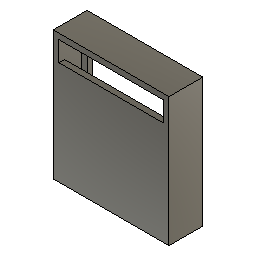
BME680_ENCLOSURE v4 (Autodesk Fusion 360 design; units mm, degrees)
Autodesk Fusion 360 part; units mm, degrees
(part 1 of 2)
sketch "Esboço1" plane through (0, 0.8, 0) normal (0, 1, 0) x (-1, 0, 0)
  line L0 (2.5, -12.15) -> (2.5, -7.85)
  arc A0 (3.5, -6.85) -> (2.5, -7.85) centre (3.5, -7.85) ccw
  line L1 (3.5, -6.85) -> (6.7, -6.85)
  line L2 (6.7, -6.85) -> (8.2, -5.35)
  line L3 (8.2, -5.35) -> (8.2, 6.85)
  line L4 (8.2, 6.85) -> (-8.2, 6.85)
  line L5 (-8.2, 6.85) -> (-8.2, -5.35)
  line L6 (-8.2, -5.35) -> (-6.7, -6.85)
  line L7 (-6.7, -6.85) -> (-3.5, -6.85)
  arc A1 (-2.5, -7.85) -> (-3.5, -6.85) centre (-3.5, -7.85) ccw
  line L8 (-2.5, -7.85) -> (-2.5, -12.15)
  line L9 (-2.5, -12.15) -> (2.5, -12.15)
  circle A2 centre (6.35, 5.85) radius 0.6
  circle A3 centre (-6.35, 5.85) radius 0.6
  circle A4 centre (-3.81, 5.85) radius 0.6
  circle A5 centre (-1.27, 5.85) radius 0.6
  circle A6 centre (1.27, 5.85) radius 0.6
  circle A7 centre (3.81, 5.85) radius 0.6
  spline S0 degree 3 poles (4.0814, 2.2721) (4.0816, 2.2764) (4.0819, 2.2848) (4.086, 2.2968) (4.0921, 2.3078) (4.1006, 2.3174) (4.1105, 2.3255) (4.1217, 2.3314) (4.1337, 2.3352) (4.1421, 2.3355) (4.1464, 2.3357) knots 0 0 0 0 0.126655 0.249859 0.371763 0.500453 0.628013 0.750799 0.873345 1 1 1 1
  spline S1 degree 3 poles (4.1464, 2.3357) (4.1506, 2.3355) (4.1588, 2.3352) (4.1707, 2.3313) (4.1818, 2.3255) (4.1915, 2.3174) (4.1998, 2.3078) (4.2056, 2.2966) (4.2095, 2.2845) (4.2098, 2.2761) (4.21, 2.2719) knots 0 0 0 0 0.12536 0.246668 0.370351 0.497111 0.625295 0.748978 0.872419 1 1 1 1
  line L10 (4.21, 2.2719) -> (4.21, 2.0201)
  spline S2 degree 3 poles (4.21, 2.0201) (4.2095, 2.0119) (4.2086, 1.9954) (4.2022, 1.9709) (4.1923, 1.9469) (4.1787, 1.9238) (4.1627, 1.9022) (4.1448, 1.8833) (4.1253, 1.8673) (4.1109, 1.8593) (4.1038, 1.8554) knots 0 0 0 0 0.120295 0.241539 0.367541 0.499794 0.632883 0.759219 0.880834 1 1 1 1
  line L11 (4.1038, 1.8554) -> (3.8515, 1.7288)
  spline S3 degree 3 poles (3.8515, 1.7288) (3.8401, 1.7233) (3.8175, 1.7125) (3.7819, 1.7011) (3.7455, 1.6941) (3.721, 1.6933) (3.7087, 1.6929) knots 0 0 0 0 0.255305 0.504536 0.751856 1 1 1 1
  spline S4 degree 3 poles (3.7087, 1.6929) (3.697, 1.6934) (3.6734, 1.6944) (3.6378, 1.702) (3.6016, 1.7137) (3.5784, 1.7251) (3.5665, 1.731) knots 0 0 0 0 0.234952 0.477147 0.731798 1 1 1 1
  line L12 (3.5665, 1.731) -> (3.3165, 1.8583)
  spline S5 degree 3 poles (3.3165, 1.8583) (3.3087, 1.8625) (3.2931, 1.8709) (3.2726, 1.8875) (3.2543, 1.9064) (3.2388, 1.9278) (3.2259, 1.951) (3.2168, 1.976) (3.2109, 2.0022) (3.2103, 2.0201) (3.21, 2.0292) knots 0 0 0 0 0.125475 0.2491 0.371934 0.496998 0.621836 0.746394 0.871303 1 1 1 1
  line L13 (3.21, 2.0292) -> (3.21, 2.2721)
  spline S6 degree 3 poles (3.21, 2.2721) (3.2102, 2.2764) (3.2106, 2.2848) (3.2143, 2.2968) (3.2205, 2.3077) (3.2287, 2.3174) (3.2384, 2.3255) (3.2493, 2.3314) (3.2612, 2.3352) (3.2694, 2.3355) (3.2736, 2.3357) knots 0 0 0 0 0.127946 0.25174 0.374887 0.503437 0.63056 0.752626 0.874282 1 1 1 1
  spline S7 degree 3 poles (3.2736, 2.3357) (3.2779, 2.3355) (3.2863, 2.3352) (3.2983, 2.3313) (3.3097, 2.3258) (3.3195, 2.3176) (3.3282, 2.3083) (3.3339, 2.2972) (3.3381, 2.2855) (3.3384, 2.2772) (3.3386, 2.273) knots 0 0 0 0 0.127432 0.250729 0.375227 0.50357 0.631371 0.752946 0.874787 1 1 1 1
  line L14 (3.3386, 2.273) -> (3.3386, 2.2071)
  line L15 (3.3386, 2.2071) -> (4.0814, 2.2071)
  line L16 (4.0814, 2.2071) -> (4.0814, 2.2721)
  spline S8 degree 3 poles (1.4325, 4.1605) (1.4397, 4.1654) (1.4537, 4.175) (1.4768, 4.1854) (1.5009, 4.1917) (1.5174, 4.1925) (1.5256, 4.1929) knots 0 0 0 0 0.259405 0.508544 0.754257 1 1 1 1
  spline S9 degree 3 poles (1.5256, 4.1929) (1.535, 4.1923) (1.5536, 4.1913) (1.5805, 4.1835) (1.6052, 4.1701) (1.6275, 4.1522) (1.6461, 4.1305) (1.6601, 4.1063) (1.6686, 4.0797) (1.6695, 4.0612) (1.67, 4.0518) knots 0 0 0 0 0.126245 0.24873 0.371883 0.501018 0.62976 0.75261 0.873755 1 1 1 1
  line L17 (1.67, 4.0518) -> (1.67, 3.729)
  spline S10 degree 3 poles (1.67, 3.729) (1.6694, 3.7192) (1.6683, 3.6993) (1.6576, 3.6704) (1.6412, 3.6426) (1.6227, 3.6208) (1.6054, 3.6047) (1.5915, 3.5937) (1.5766, 3.5849) (1.5613, 3.5772) (1.5452, 3.5713) (1.5284, 3.5674) (1.5109, 3.5648) (1.499, 3.5645) (1.493, 3.5643) knots 0 0 0 0 0.110459 0.223148 0.342644 0.474148 0.54296 0.6087 0.673406 0.737899 0.801293 0.865961 0.932005 1 1 1 1
  spline S11 degree 3 poles (1.493, 3.5643) (1.4886, 3.5646) (1.4799, 3.5651) (1.4673, 3.5689) (1.456, 3.5759) (1.4461, 3.5851) (1.4377, 3.5955) (1.4315, 3.6069) (1.4277, 3.619) (1.4273, 3.6273) (1.4271, 3.6315) knots 0 0 0 0 0.127348 0.250965 0.376177 0.506901 0.638364 0.760387 0.87927 1 1 1 1
  spline S12 degree 3 poles (1.4271, 3.6315) (1.4273, 3.6369) (1.4275, 3.6469) (1.4303, 3.6607) (1.4352, 3.6717) (1.4423, 3.6806) (1.4526, 3.6868) (1.4652, 3.6929) (1.4814, 3.6983) (1.4996, 3.7029) (1.5174, 3.7084) (1.5315, 3.7187) (1.54, 3.7328) (1.541, 3.7434) (1.5414, 3.7489) knots 0 0 0 0 0.089812 0.165231 0.230095 0.287663 0.349673 0.426046 0.519675 0.62936 0.736624 0.826058 0.910331 1 1 1 1
  line L18 (1.5414, 3.7489) -> (1.5414, 4.0431)
  spline S13 degree 3 poles (1.5414, 4.0431) (1.5414, 4.0462) (1.5412, 4.0518) (1.5382, 4.0588) (1.5333, 4.0637) (1.529, 4.0641) (1.5267, 4.0643) knots 0 0 0 0 0.323315 0.566859 0.773057 1 1 1 1
  spline S14 degree 3 poles (1.5267, 4.0643) (1.5233, 4.0639) (1.5155, 4.0631) (1.5091, 4.0583) (1.5055, 4.0556) knots 0 0 0 0 0.42835 1 1 1 1
  line L19 (1.5055, 4.0556) -> (0.9075, 3.5973)
  spline S15 degree 3 poles (0.9075, 3.5973) (0.9003, 3.5922) (0.8862, 3.5822) (0.8627, 3.5721) (0.8385, 3.5653) (0.8221, 3.5646) (0.8137, 3.5643) knots 0 0 0 0 0.261351 0.512303 0.754244 1 1 1 1
  spline S16 degree 3 poles (0.8137, 3.5643) (0.8045, 3.5647) (0.7861, 3.5656) (0.7596, 3.5735) (0.735, 3.5863) (0.7129, 3.6038) (0.6942, 3.6241) (0.68, 3.6461) (0.6716, 3.6698) (0.6705, 3.6861) (0.67, 3.6942) knots 0 0 0 0 0.130284 0.257797 0.385118 0.519315 0.651174 0.771096 0.886275 1 1 1 1
  line L20 (0.67, 3.6942) -> (0.67, 4.0283)
  spline S17 degree 3 poles (0.67, 4.0283) (0.6702, 4.0338) (0.6706, 4.0446) (0.6731, 4.0604) (0.6771, 4.0758) (0.6829, 4.0906) (0.6906, 4.1047) (0.6998, 4.1184) (0.7105, 4.1316) (0.727, 4.1479) (0.7492, 4.1656) (0.7781, 4.1813) (0.8085, 4.1911) (0.8294, 4.1923) (0.8399, 4.1929) knots 0 0 0 0 0.062642 0.124202 0.184472 0.245252 0.306591 0.369566 0.434735 0.502591 0.635605 0.760198 0.879447 1 1 1 1
  spline S18 degree 3 poles (0.8399, 4.1929) (0.8456, 4.1927) (0.8564, 4.1923) (0.8714, 4.1891) (0.8843, 4.1841) (0.8947, 4.1765) (0.9032, 4.1671) (0.9089, 4.1552) (0.9123, 4.1414) (0.9127, 4.1316) (0.9129, 4.1263) knots 0 0 0 0 0.152342 0.285545 0.405068 0.516839 0.624561 0.739342 0.861447 1 1 1 1
  spline S19 degree 3 poles (0.9129, 4.1263) (0.9127, 4.1222) (0.9123, 4.114) (0.9083, 4.1024) (0.9023, 4.0916) (0.8939, 4.0823) (0.8839, 4.0742) (0.8728, 4.0685) (0.8607, 4.0649) (0.8524, 4.0645) (0.8481, 4.0643) knots 0 0 0 0 0.123971 0.246778 0.365389 0.494204 0.623565 0.750071 0.871557 1 1 1 1
  spline S20 degree 3 poles (0.8481, 4.0643) (0.8447, 4.0641) (0.8381, 4.0638) (0.8286, 4.0612) (0.8201, 4.057) (0.8127, 4.0511) (0.8063, 4.044) (0.8019, 4.0357) (0.799, 4.0266) (0.7987, 4.0203) (0.7986, 4.017) knots 0 0 0 0 0.13474 0.258614 0.382591 0.505187 0.629267 0.752001 0.871073 1 1 1 1
  line L21 (0.7986, 4.017) -> (0.7986, 3.7125)
  spline S21 degree 3 poles (0.7986, 3.7125) (0.7986, 3.7095) (0.7987, 3.7043) (0.8021, 3.6977) (0.8076, 3.6931) (0.8122, 3.693) (0.8146, 3.6929) knots 0 0 0 0 0.302016 0.536312 0.750494 1 1 1 1
  spline S22 degree 3 poles (0.8146, 3.6929) (0.8176, 3.6933) (0.825, 3.6945) (0.8308, 3.6992) (0.8343, 3.702) knots 0 0 0 0 0.406145 1 1 1 1
  line L22 (0.8343, 3.702) -> (1.4325, 4.1605)
  line L23 (1.095, 3.1161) -> (0.8374, 2.983)
  spline S23 degree 3 poles (0.8374, 2.983) (0.8313, 2.9797) (0.8198, 2.9734) (0.8069, 2.9586) (0.7993, 2.9405) (0.7988, 2.9274) (0.7986, 2.9205) knots 0 0 0 0 0.262753 0.501306 0.739158 1 1 1 1
  line L24 (0.7986, 2.9205) -> (0.7986, 2.6875)
  spline S24 degree 3 poles (0.7986, 2.6875) (0.7984, 2.6832) (0.798, 2.6746) (0.7942, 2.6624) (0.7884, 2.6509) (0.78, 2.6409) (0.7705, 2.632) (0.7592, 2.6261) (0.7472, 2.6219) (0.7386, 2.6216) (0.7343, 2.6214) knots 0 0 0 0 0.126957 0.249782 0.372684 0.501426 0.62965 0.751659 0.873043 1 1 1 1
  spline S25 degree 3 poles (0.7343, 2.6214) (0.7299, 2.6216) (0.7214, 2.6219) (0.7094, 2.6261) (0.6981, 2.632) (0.6886, 2.6409) (0.6801, 2.6507) (0.6744, 2.6621) (0.6705, 2.6742) (0.6702, 2.6827) (0.67, 2.6871) knots 0 0 0 0 0.127439 0.249283 0.371755 0.500466 0.627999 0.751368 0.872561 1 1 1 1
  line L25 (0.67, 2.6871) -> (0.67, 2.927)
  spline S26 degree 3 poles (0.67, 2.927) (0.6703, 2.9348) (0.671, 2.9506) (0.6771, 2.9743) (0.6863, 2.9983) (0.6988, 3.022) (0.7133, 3.044) (0.729, 3.063) (0.7454, 3.0786) (0.7577, 3.086) (0.7635, 3.0895) knots 0 0 0 0 0.119524 0.243206 0.374508 0.515457 0.654341 0.779636 0.894797 1 1 1 1
  line L26 (0.7635, 3.0895) -> (1.0454, 3.235)
  spline S27 degree 3 poles (1.0454, 3.235) (1.0556, 3.2395) (1.0755, 3.2484) (1.1068, 3.2574) (1.1384, 3.2633) (1.1596, 3.264) (1.1702, 3.2643) knots 0 0 0 0 0.256397 0.506809 0.754246 1 1 1 1
  spline S28 degree 3 poles (1.1702, 3.2643) (1.1816, 3.2639) (1.2038, 3.2633) (1.2359, 3.2581) (1.2657, 3.2496) (1.2839, 3.2409) (1.2928, 3.2366) knots 0 0 0 0 0.269644 0.524554 0.766799 1 1 1 1
  line L27 (1.2928, 3.2366) -> (1.5718, 3.0895)
  spline S29 degree 3 poles (1.5718, 3.0895) (1.5782, 3.0857) (1.5913, 3.0779) (1.609, 3.0625) (1.6258, 3.0446) (1.6409, 3.0241) (1.6537, 3.0024) (1.6629, 2.9804) (1.669, 2.9587) (1.6697, 2.9443) (1.67, 2.9373) knots 0 0 0 0 0.119157 0.241726 0.37148 0.508504 0.645292 0.77099 0.888372 1 1 1 1
  line L28 (1.67, 2.9373) -> (1.67, 2.6853)
  spline S30 degree 3 poles (1.67, 2.6853) (1.6698, 2.681) (1.6695, 2.6726) (1.6657, 2.6606) (1.6598, 2.6496) (1.6515, 2.64) (1.6418, 2.6316) (1.6307, 2.6258) (1.6188, 2.622) (1.6106, 2.6216) (1.6064, 2.6214) knots 0 0 0 0 0.12765 0.251158 0.372942 0.501195 0.629448 0.753198 0.874572 1 1 1 1
  spline S31 degree 3 poles (1.6064, 2.6214) (1.6021, 2.6216) (1.5937, 2.622) (1.5817, 2.6258) (1.5705, 2.6316) (1.5606, 2.64) (1.552, 2.6496) (1.546, 2.6608) (1.5419, 2.6728) (1.5416, 2.6812) (1.5414, 2.6855) knots 0 0 0 0 0.126235 0.248374 0.370753 0.49928 0.627542 0.75097 0.873765 1 1 1 1
  line L29 (1.5414, 2.6855) -> (1.5414, 2.9299)
  spline S32 degree 3 poles (1.5414, 2.9299) (1.5413, 2.9348) (1.5409, 2.9446) (1.534, 2.9584) (1.5227, 2.9704) (1.5128, 2.9762) (1.5075, 2.9792) knots 0 0 0 0 0.230337 0.460431 0.709763 1 1 1 1
  line L30 (1.5075, 2.9792) -> (1.245, 3.1181)
  spline S33 degree 3 poles (1.245, 3.1181) (1.2397, 3.1207) (1.2289, 3.126) (1.2112, 3.1312) (1.1922, 3.1346) (1.1792, 3.1353) (1.1725, 3.1357) knots 0 0 0 0 0.234765 0.479498 0.732423 1 1 1 1
  spline S34 degree 3 poles (1.1725, 3.1357) (1.1654, 3.1352) (1.1516, 3.1341) (1.1315, 3.1304) (1.1126, 3.1243) (1.1008, 3.1188) (1.095, 3.1161) knots 0 0 0 0 0.264576 0.515798 0.760431 1 1 1 1
  spline S35 degree 3 poles (0.7343, 1.7214) (0.7299, 1.7216) (0.7215, 1.7219) (0.7094, 1.7258) (0.6982, 1.7316) (0.6885, 1.7397) (0.6802, 1.7491) (0.6744, 1.7599) (0.6705, 1.7715) (0.6702, 1.7796) (0.67, 1.7837) knots 0 0 0 0 0.130816 0.255221 0.37987 0.50762 0.635092 0.755789 0.875899 1 1 1 1
  line L31 (0.67, 1.7837) -> (0.67, 2.3357)
  line L32 (0.67, 2.3357) -> (1.6068, 2.3357)
  spline S36 degree 3 poles (1.6068, 2.3357) (1.6109, 2.3355) (1.6191, 2.3351) (1.6309, 2.3314) (1.6418, 2.3252) (1.6516, 2.317) (1.6598, 2.3071) (1.6656, 2.296) (1.6695, 2.284) (1.6698, 2.2757) (1.67, 2.2714) knots 0 0 0 0 0.123399 0.244963 0.368017 0.496471 0.626642 0.750586 0.87215 1 1 1 1
  spline S37 degree 3 poles (1.67, 2.2714) (1.6698, 2.2672) (1.6695, 2.2588) (1.6656, 2.2469) (1.6599, 2.2357) (1.6514, 2.2261) (1.6419, 2.2176) (1.631, 2.2115) (1.6193, 2.2077) (1.6112, 2.2073) (1.6071, 2.2071) knots 0 0 0 0 0.128158 0.250015 0.374257 0.50302 0.633235 0.756586 0.876304 1 1 1 1
  line L33 (1.6071, 2.2071) -> (0.7986, 2.2071)
  line L34 (0.7986, 2.2071) -> (0.7986, 1.7828)
  spline S38 degree 3 poles (0.7986, 1.7828) (0.7984, 1.7788) (0.798, 1.7708) (0.7941, 1.7594) (0.7884, 1.7487) (0.78, 1.7395) (0.7703, 1.7314) (0.7593, 1.7255) (0.7471, 1.722) (0.7386, 1.7216) (0.7343, 1.7214) knots 0 0 0 0 0.122686 0.24145 0.362962 0.489589 0.618201 0.743691 0.868301 1 1 1 1
  spline S39 degree 3 poles (4.1455, 2.7786) (4.1498, 2.7784) (4.1582, 2.7781) (4.1702, 2.7739) (4.1815, 2.7682) (4.1912, 2.7596) (4.1996, 2.7497) (4.2056, 2.7384) (4.2095, 2.7263) (4.2098, 2.7179) (4.21, 2.7136) knots 0 0 0 0 0.12578 0.248133 0.370071 0.499543 0.627607 0.75252 0.87422 1 1 1 1
  spline S40 degree 3 poles (4.21, 2.7136) (4.2098, 2.7093) (4.2094, 2.7009) (4.2057, 2.689) (4.1997, 2.6779) (4.1915, 2.6682) (4.1815, 2.6603) (4.1704, 2.6543) (4.1582, 2.6506) (4.1496, 2.6502) (4.1453, 2.65) knots 0 0 0 0 0.126508 0.248912 0.369606 0.496712 0.624124 0.746767 0.871289 1 1 1 1
  line L35 (4.1453, 2.65) -> (3.21, 2.65)
  line L36 (3.21, 2.65) -> (3.21, 2.8234)
  line L37 (3.21, 2.8234) -> (3.9814, 3.1357)
  line L38 (3.9814, 3.1357) -> (3.2727, 3.1357)
  spline S41 degree 3 poles (3.2727, 3.1357) (3.2685, 3.1359) (3.2603, 3.1363) (3.2485, 3.1401) (3.2375, 3.1459) (3.2281, 3.1543) (3.22, 3.164) (3.2141, 3.175) (3.2106, 3.1872) (3.2102, 3.1957) (3.21, 3.2) knots 0 0 0 0 0.12562 0.24718 0.36915 0.495897 0.622919 0.746859 0.869929 1 1 1 1
  spline S42 degree 3 poles (3.21, 3.2) (3.2102, 3.2043) (3.2105, 3.2128) (3.2144, 3.2249) (3.2202, 3.2361) (3.2283, 3.2457) (3.2377, 3.2541) (3.2487, 3.2599) (3.2606, 3.2638) (3.2689, 3.2641) (3.2732, 3.2643) knots 0 0 0 0 0.129701 0.253047 0.376633 0.503294 0.629681 0.751304 0.872518 1 1 1 1
  line L39 (3.2732, 3.2643) -> (4.21, 3.2643)
  line L40 (4.21, 3.2643) -> (4.21, 3.0908)
  line L41 (4.21, 3.0908) -> (3.4386, 2.7786)
  line L42 (3.4386, 2.7786) -> (4.1455, 2.7786)
  line L43 (3.91, 4.144) -> (4.1453, 3.9634)
  spline S43 degree 3 poles (4.1453, 3.9634) (4.1497, 3.9599) (4.1587, 3.9528) (4.1707, 3.94) (4.1816, 3.9253) (4.1916, 3.9093) (4.1999, 3.8921) (4.2056, 3.8741) (4.2094, 3.8559) (4.2098, 3.8436) (4.21, 3.8375) knots 0 0 0 0 0.114743 0.234412 0.358473 0.489173 0.620749 0.748955 0.874792 1 1 1 1
  line L44 (4.21, 3.8375) -> (4.21, 3.6384)
  spline S44 degree 3 poles (4.21, 3.6384) (4.2098, 3.6344) (4.2094, 3.6265) (4.2057, 3.6153) (4.1997, 3.605) (4.1916, 3.5959) (4.1821, 3.5881) (4.171, 3.5827) (4.159, 3.5792) (4.1507, 3.5788) (4.1464, 3.5786) knots 0 0 0 0 0.122534 0.243369 0.362993 0.48858 0.61799 0.741514 0.868297 1 1 1 1
  spline S45 degree 3 poles (4.1464, 3.5786) (4.1419, 3.5788) (4.1331, 3.5791) (4.1207, 3.5828) (4.1094, 3.5887) (4.0998, 3.597) (4.0919, 3.6064) (4.0858, 3.6165) (4.082, 3.627) (4.0816, 3.6343) (4.0814, 3.6379) knots 0 0 0 0 0.138236 0.26975 0.397109 0.529103 0.657862 0.775204 0.889197 1 1 1 1
  line L45 (4.0814, 3.6379) -> (4.0814, 3.8263)
  spline S46 degree 3 poles (4.0814, 3.8263) (4.0807, 3.8309) (4.0792, 3.84) (4.0727, 3.8528) (4.0635, 3.8648) (4.0555, 3.8714) (4.0513, 3.8748) knots 0 0 0 0 0.233592 0.47014 0.725097 1 1 1 1
  line L46 (4.0513, 3.8748) -> (3.8288, 4.0433)
  spline S47 degree 3 poles (3.8287, 4.0433) (3.824, 4.0467) (3.8141, 4.0536) (3.7962, 4.0598) (3.776, 4.0639) (3.7616, 4.0642) (3.754, 4.0643) knots 0 0 0 0 0.220731 0.452888 0.711856 1 1 1 1
  line L47 (3.754, 4.0643) -> (3.4033, 4.0643)
  spline S48 degree 3 poles (3.4033, 4.0643) (3.399, 4.0641) (3.3905, 4.0636) (3.3782, 4.0605) (3.3671, 4.055) (3.3573, 4.0474) (3.3492, 4.0384) (3.3428, 4.0283) (3.3391, 4.0171) (3.3388, 4.0093) (3.3386, 4.0054) knots 0 0 0 0 0.133582 0.261589 0.386788 0.514383 0.641108 0.759565 0.877845 1 1 1 1
  line L48 (3.3386, 4.0054) -> (3.3386, 3.7661)
  spline S49 degree 3 poles (3.3386, 3.7661) (3.3388, 3.7622) (3.3391, 3.7545) (3.3429, 3.7435) (3.3489, 3.7334) (3.3572, 3.7245) (3.3667, 3.7166) (3.3777, 3.7114) (3.3894, 3.7077) (3.3975, 3.7073) (3.4017, 3.7071) knots 0 0 0 0 0.12193 0.240024 0.359311 0.488213 0.619439 0.744696 0.868774 1 1 1 1
  line L49 (3.4017, 3.7071) -> (3.5386, 3.7071)
  line L50 (3.5386, 3.7071) -> (3.5386, 3.8324)
  spline S50 degree 3 poles (3.5386, 3.8324) (3.5387, 3.8366) (3.5391, 3.8447) (3.543, 3.8562) (3.5487, 3.8669) (3.5571, 3.8759) (3.5668, 3.8836) (3.578, 3.889) (3.5901, 3.8922) (3.5985, 3.8926) (3.6029, 3.8929) knots 0 0 0 0 0.12753 0.24661 0.368445 0.493715 0.619846 0.743608 0.867951 1 1 1 1
  spline S51 degree 3 poles (3.6029, 3.8929) (3.6072, 3.8927) (3.6157, 3.8923) (3.6277, 3.8887) (3.639, 3.8834) (3.6486, 3.8754) (3.657, 3.8662) (3.6628, 3.8553) (3.6666, 3.8434) (3.667, 3.8351) (3.6671, 3.8308) knots 0 0 0 0 0.130449 0.253876 0.376138 0.502122 0.627547 0.749871 0.871784 1 1 1 1
  line L51 (3.6671, 3.8308) -> (3.6671, 3.5786)
  line L52 (3.6671, 3.5786) -> (3.4013, 3.5786)
  spline S52 degree 3 poles (3.4013, 3.5786) (3.3948, 3.5788) (3.382, 3.5791) (3.3632, 3.5816) (3.3453, 3.5859) (3.3279, 3.5916) (3.3114, 3.5993) (3.2954, 3.6085) (3.2803, 3.6195) (3.266, 3.632) (3.2531, 3.6456) (3.2415, 3.66) (3.2317, 3.6751) (3.2238, 3.691) (3.2174, 3.7075) (3.2133, 3.7249) (3.2105, 3.7428) (3.2102, 3.755) (3.21, 3.7612) knots 0 0 0 0 0.066145 0.130486 0.192935 0.254659 0.316509 0.378777 0.442433 0.507021 0.572022 0.634174 0.695688 0.755127 0.815217 0.875451 0.93689 1 1 1 1
  line L53 (3.21, 3.7612) -> (3.21, 4.0089)
  spline S53 degree 3 poles (3.21, 4.0089) (3.2102, 4.0151) (3.2105, 4.0274) (3.2133, 4.0454) (3.2174, 4.0628) (3.2239, 4.0794) (3.2316, 4.0955) (3.2413, 4.1108) (3.2528, 4.1254) (3.2659, 4.139) (3.28, 4.1517) (3.295, 4.1628) (3.3109, 4.1718) (3.3274, 4.1796) (3.3446, 4.1856) (3.3625, 4.1898) (3.3811, 4.1923) (3.3938, 4.1927) (3.4002, 4.1929) knots 0 0 0 0 0.063095 0.12527 0.185491 0.245567 0.306354 0.367444 0.430177 0.495163 0.560238 0.623265 0.685519 0.746665 0.808622 0.871056 0.934629 1 1 1 1
  line L54 (3.4002, 4.1929) -> (3.7513, 4.1929)
  spline S54 degree 3 poles (3.7513, 4.1929) (3.759, 4.1928) (3.7742, 4.1926) (3.7964, 4.1899) (3.8177, 4.1863) (3.8381, 4.1809) (3.8575, 4.1739) (3.8762, 4.1658) (3.8936, 4.1556) (3.9046, 4.1479) (3.91, 4.144) knots 0 0 0 0 0.137364 0.268874 0.396291 0.520543 0.642479 0.762456 0.881345 1 1 1 1
  line L55 (6.175, 2.1875) -> (5.9174, 2.0545)
  spline S55 degree 3 poles (5.9174, 2.0545) (5.9113, 2.0512) (5.8998, 2.0449) (5.8869, 2.03) (5.8793, 2.0119) (5.8788, 1.9988) (5.8786, 1.992) knots 0 0 0 0 0.262753 0.501306 0.739158 1 1 1 1
  line L56 (5.8786, 1.992) -> (5.8786, 1.7589)
  spline S56 degree 3 poles (5.8786, 1.7589) (5.8784, 1.7546) (5.878, 1.746) (5.8742, 1.7338) (5.8684, 1.7223) (5.86, 1.7123) (5.8505, 1.7035) (5.8392, 1.6975) (5.8272, 1.6933) (5.8186, 1.693) (5.8143, 1.6929) knots 0 0 0 0 0.126957 0.249782 0.372684 0.501426 0.62965 0.751659 0.873043 1 1 1 1
  spline S57 degree 3 poles (5.8143, 1.6929) (5.8099, 1.693) (5.8014, 1.6933) (5.7894, 1.6975) (5.7781, 1.7035) (5.7686, 1.7123) (5.7601, 1.7221) (5.7544, 1.7335) (5.7505, 1.7457) (5.7502, 1.7541) (5.75, 1.7585) knots 0 0 0 0 0.127439 0.249283 0.371755 0.500466 0.627999 0.751368 0.872561 1 1 1 1
  line L57 (5.75, 1.7585) -> (5.75, 1.9984)
  spline S58 degree 3 poles (5.75, 1.9984) (5.7503, 2.0062) (5.751, 2.022) (5.7571, 2.0457) (5.7663, 2.0698) (5.7788, 2.0934) (5.7933, 2.1154) (5.809, 2.1344) (5.8254, 2.15) (5.8377, 2.1574) (5.8435, 2.1609) knots 0 0 0 0 0.119524 0.243206 0.374508 0.515457 0.654341 0.779636 0.894797 1 1 1 1
  line L58 (5.8435, 2.1609) -> (6.1254, 2.3065)
  spline S59 degree 3 poles (6.1254, 2.3065) (6.1356, 2.311) (6.1555, 2.3198) (6.1868, 2.3288) (6.2184, 2.3347) (6.2396, 2.3354) (6.2502, 2.3357) knots 0 0 0 0 0.256397 0.506809 0.754246 1 1 1 1
  spline S60 degree 3 poles (6.2502, 2.3357) (6.2616, 2.3354) (6.2838, 2.3347) (6.3159, 2.3295) (6.3457, 2.321) (6.3639, 2.3123) (6.3728, 2.308) knots 0 0 0 0 0.269644 0.524554 0.766799 1 1 1 1
  line L59 (6.3728, 2.308) -> (6.6518, 2.1609)
  spline S61 degree 3 poles (6.6518, 2.1609) (6.6582, 2.1571) (6.6713, 2.1493) (6.689, 2.1339) (6.7058, 2.1161) (6.7209, 2.0956) (6.7337, 2.0739) (6.7429, 2.0518) (6.749, 2.0302) (6.7497, 2.0157) (6.75, 2.0087) knots 0 0 0 0 0.119157 0.241726 0.37148 0.508504 0.645292 0.77099 0.888372 1 1 1 1
  line L60 (6.75, 2.0087) -> (6.75, 1.7567)
  spline S62 degree 3 poles (6.75, 1.7567) (6.7498, 1.7524) (6.7495, 1.744) (6.7457, 1.732) (6.7398, 1.721) (6.7315, 1.7114) (6.7218, 1.703) (6.7107, 1.6973) (6.6988, 1.6934) (6.6906, 1.693) (6.6864, 1.6929) knots 0 0 0 0 0.12765 0.251158 0.372942 0.501195 0.629448 0.753198 0.874572 1 1 1 1
  spline S63 degree 3 poles (6.6864, 1.6929) (6.6821, 1.693) (6.6737, 1.6934) (6.6617, 1.6972) (6.6505, 1.7031) (6.6406, 1.7114) (6.632, 1.721) (6.626, 1.7322) (6.6219, 1.7442) (6.6216, 1.7526) (6.6214, 1.7569) knots 0 0 0 0 0.126235 0.248374 0.370753 0.49928 0.627542 0.75097 0.873765 1 1 1 1
  line L61 (6.6214, 1.7569) -> (6.6214, 2.0013)
  spline S64 degree 3 poles (6.6214, 2.0013) (6.6213, 2.0063) (6.6209, 2.0161) (6.614, 2.0298) (6.6027, 2.0418) (6.5928, 2.0476) (6.5875, 2.0507) knots 0 0 0 0 0.230337 0.460431 0.709763 1 1 1 1
  line L62 (6.5875, 2.0507) -> (6.325, 2.1895)
  spline S65 degree 3 poles (6.325, 2.1895) (6.3197, 2.1921) (6.3089, 2.1975) (6.2912, 2.2026) (6.2722, 2.206) (6.2592, 2.2068) (6.2525, 2.2071) knots 0 0 0 0 0.234765 0.479498 0.732423 1 1 1 1
  spline S66 degree 3 poles (6.2525, 2.2071) (6.2454, 2.2066) (6.2316, 2.2056) (6.2115, 2.2018) (6.1926, 2.1957) (6.1808, 2.1902) (6.175, 2.1875) knots 0 0 0 0 0.264576 0.515798 0.760431 1 1 1 1
  line L63 (6.175, 3.1161) -> (5.9174, 2.983)
  spline S67 degree 3 poles (5.9174, 2.983) (5.9113, 2.9797) (5.8998, 2.9734) (5.8869, 2.9586) (5.8793, 2.9405) (5.8788, 2.9274) (5.8786, 2.9205) knots 0 0 0 0 0.262753 0.501306 0.739158 1 1 1 1
  line L64 (5.8786, 2.9205) -> (5.8786, 2.6875)
  spline S68 degree 3 poles (5.8786, 2.6875) (5.8784, 2.6832) (5.878, 2.6746) (5.8742, 2.6624) (5.8684, 2.6509) (5.86, 2.6409) (5.8505, 2.632) (5.8392, 2.6261) (5.8272, 2.6219) (5.8186, 2.6216) (5.8143, 2.6214) knots 0 0 0 0 0.126957 0.249782 0.372684 0.501426 0.62965 0.751659 0.873043 1 1 1 1
  spline S69 degree 3 poles (5.8143, 2.6214) (5.8099, 2.6216) (5.8014, 2.6219) (5.7894, 2.6261) (5.7781, 2.632) (5.7686, 2.6409) (5.7601, 2.6507) (5.7544, 2.6621) (5.7505, 2.6742) (5.7502, 2.6827) (5.75, 2.6871) knots 0 0 0 0 0.127439 0.249283 0.371755 0.500466 0.627999 0.751368 0.872561 1 1 1 1
  line L65 (5.75, 2.6871) -> (5.75, 2.927)
  spline S70 degree 3 poles (5.75, 2.927) (5.7503, 2.9348) (5.751, 2.9506) (5.7571, 2.9743) (5.7663, 2.9983) (5.7788, 3.022) (5.7933, 3.044) (5.809, 3.063) (5.8254, 3.0786) (5.8377, 3.086) (5.8435, 3.0895) knots 0 0 0 0 0.119524 0.243206 0.374508 0.515457 0.654341 0.779636 0.894797 1 1 1 1
  line L66 (5.8435, 3.0895) -> (6.1254, 3.235)
  spline S71 degree 3 poles (6.1254, 3.235) (6.1356, 3.2395) (6.1555, 3.2484) (6.1868, 3.2574) (6.2184, 3.2633) (6.2396, 3.264) (6.2502, 3.2643) knots 0 0 0 0 0.256397 0.506809 0.754246 1 1 1 1
  spline S72 degree 3 poles (6.2502, 3.2643) (6.2616, 3.2639) (6.2838, 3.2633) (6.3159, 3.2581) (6.3457, 3.2496) (6.3639, 3.2409) (6.3728, 3.2366) knots 0 0 0 0 0.269644 0.524554 0.766799 1 1 1 1
  line L67 (6.3728, 3.2366) -> (6.6518, 3.0895)
  spline S73 degree 3 poles (6.6518, 3.0895) (6.6582, 3.0857) (6.6713, 3.0779) (6.689, 3.0625) (6.7058, 3.0446) (6.7209, 3.0241) (6.7337, 3.0024) (6.7429, 2.9804) (6.749, 2.9587) (6.7497, 2.9443) (6.75, 2.9373) knots 0 0 0 0 0.119157 0.241726 0.37148 0.508504 0.645292 0.77099 0.888372 1 1 1 1
  line L68 (6.75, 2.9373) -> (6.75, 2.6853)
  spline S74 degree 3 poles (6.75, 2.6853) (6.7498, 2.681) (6.7495, 2.6726) (6.7457, 2.6606) (6.7398, 2.6496) (6.7315, 2.64) (6.7218, 2.6316) (6.7107, 2.6258) (6.6988, 2.622) (6.6906, 2.6216) (6.6864, 2.6214) knots 0 0 0 0 0.12765 0.251158 0.372942 0.501195 0.629448 0.753198 0.874572 1 1 1 1
  spline S75 degree 3 poles (6.6864, 2.6214) (6.6821, 2.6216) (6.6737, 2.622) (6.6617, 2.6258) (6.6505, 2.6316) (6.6406, 2.64) (6.632, 2.6496) (6.626, 2.6608) (6.6219, 2.6728) (6.6216, 2.6812) (6.6214, 2.6855) knots 0 0 0 0 0.126235 0.248374 0.370753 0.49928 0.627542 0.75097 0.873765 1 1 1 1
  line L69 (6.6214, 2.6855) -> (6.6214, 2.9299)
  spline S76 degree 3 poles (6.6214, 2.9299) (6.6213, 2.9348) (6.6209, 2.9446) (6.614, 2.9584) (6.6027, 2.9704) (6.5928, 2.9762) (6.5875, 2.9792) knots 0 0 0 0 0.230337 0.460431 0.709763 1 1 1 1
  line L70 (6.5875, 2.9792) -> (6.325, 3.1181)
  spline S77 degree 3 poles (6.325, 3.1181) (6.3197, 3.1207) (6.3089, 3.126) (6.2912, 3.1312) (6.2722, 3.1346) (6.2592, 3.1353) (6.2525, 3.1357) knots 0 0 0 0 0.234765 0.479498 0.732423 1 1 1 1
  spline S78 degree 3 poles (6.2525, 3.1357) (6.2454, 3.1352) (6.2316, 3.1341) (6.2115, 3.1304) (6.1926, 3.1243) (6.1808, 3.1188) (6.175, 3.1161) knots 0 0 0 0 0.264576 0.515798 0.760431 1 1 1 1
  spline S79 degree 3 poles (-6.1875, 3.2319) (-6.1803, 3.2368) (-6.1663, 3.2465) (-6.1432, 3.2569) (-6.1191, 3.2631) (-6.1026, 3.2639) (-6.0944, 3.2643) knots 0 0 0 0 0.259405 0.508544 0.754257 1 1 1 1
  spline S80 degree 3 poles (-6.0944, 3.2643) (-6.085, 3.2637) (-6.0664, 3.2627) (-6.0395, 3.2549) (-6.0148, 3.2415) (-5.9925, 3.2237) (-5.9739, 3.202) (-5.9599, 3.1778) (-5.9514, 3.1511) (-5.9505, 3.1326) (-5.95, 3.1232) knots 0 0 0 0 0.126245 0.24873 0.371883 0.501018 0.62976 0.75261 0.873755 1 1 1 1
  line L71 (-5.95, 3.1232) -> (-5.95, 2.8004)
  spline S81 degree 3 poles (-5.95, 2.8004) (-5.9506, 2.7906) (-5.9517, 2.7707) (-5.9624, 2.7419) (-5.9788, 2.714) (-5.9973, 2.6922) (-6.0146, 2.6761) (-6.0285, 2.6651) (-6.0434, 2.6563) (-6.0587, 2.6486) (-6.0748, 2.6427) (-6.0916, 2.6388) (-6.1091, 2.6363) (-6.121, 2.6359) (-6.127, 2.6357) knots 0 0 0 0 0.110459 0.223148 0.342644 0.474148 0.54296 0.6087 0.673406 0.737899 0.801293 0.865961 0.932005 1 1 1 1
  spline S82 degree 3 poles (-6.127, 2.6357) (-6.1314, 2.636) (-6.1401, 2.6365) (-6.1527, 2.6404) (-6.164, 2.6473) (-6.1739, 2.6565) (-6.1823, 2.6669) (-6.1885, 2.6783) (-6.1923, 2.6904) (-6.1927, 2.6987) (-6.1929, 2.7029) knots 0 0 0 0 0.127348 0.250965 0.376177 0.506901 0.638364 0.760387 0.87927 1 1 1 1
  spline S83 degree 3 poles (-6.1929, 2.7029) (-6.1927, 2.7083) (-6.1925, 2.7184) (-6.1897, 2.7321) (-6.1848, 2.7432) (-6.1777, 2.752) (-6.1674, 2.7582) (-6.1548, 2.7643) (-6.1386, 2.7697) (-6.1204, 2.7744) (-6.1026, 2.7798) (-6.0885, 2.7901) (-6.08, 2.8042) (-6.079, 2.8148) (-6.0786, 2.8203) knots 0 0 0 0 0.089812 0.165231 0.230095 0.287663 0.349673 0.426046 0.519675 0.62936 0.736624 0.826058 0.910331 1 1 1 1
  line L72 (-6.0786, 2.8203) -> (-6.0786, 3.1145)
  spline S84 degree 3 poles (-6.0786, 3.1145) (-6.0786, 3.1177) (-6.0788, 3.1232) (-6.0818, 3.1303) (-6.0867, 3.1351) (-6.091, 3.1355) (-6.0933, 3.1357) knots 0 0 0 0 0.323315 0.566859 0.773057 1 1 1 1
  spline S85 degree 3 poles (-6.0933, 3.1357) (-6.0967, 3.1354) (-6.1045, 3.1345) (-6.1109, 3.1297) (-6.1145, 3.127) knots 0 0 0 0 0.42835 1 1 1 1
  line L73 (-6.1145, 3.127) -> (-6.7125, 2.6687)
  spline S86 degree 3 poles (-6.7125, 2.6687) (-6.7197, 2.6636) (-6.7338, 2.6536) (-6.7573, 2.6436) (-6.7815, 2.6367) (-6.7979, 2.6361) (-6.8063, 2.6357) knots 0 0 0 0 0.261351 0.512303 0.754244 1 1 1 1
  spline S87 degree 3 poles (-6.8063, 2.6357) (-6.8155, 2.6362) (-6.8339, 2.637) (-6.8604, 2.645) (-6.885, 2.6578) (-6.9071, 2.6752) (-6.9258, 2.6955) (-6.94, 2.7175) (-6.9484, 2.7412) (-6.9495, 2.7575) (-6.95, 2.7656) knots 0 0 0 0 0.130284 0.257797 0.385118 0.519315 0.651174 0.771096 0.886275 1 1 1 1
  line L74 (-6.95, 2.7656) -> (-6.95, 3.0998)
  spline S88 degree 3 poles (-6.95, 3.0998) (-6.9498, 3.1052) (-6.9494, 3.116) (-6.9469, 3.1319) (-6.9429, 3.1472) (-6.9371, 3.162) (-6.9294, 3.1761) (-6.9202, 3.1898) (-6.9095, 3.2031) (-6.893, 3.2193) (-6.8708, 3.237) (-6.8419, 3.2527) (-6.8115, 3.2625) (-6.7906, 3.2637) (-6.7801, 3.2643) knots 0 0 0 0 0.062642 0.124202 0.184472 0.245252 0.306591 0.369566 0.434735 0.502591 0.635605 0.760198 0.879447 1 1 1 1
  spline S89 degree 3 poles (-6.7801, 3.2643) (-6.7744, 3.2641) (-6.7636, 3.2637) (-6.7486, 3.2606) (-6.7357, 3.2555) (-6.7253, 3.248) (-6.7168, 3.2385) (-6.7111, 3.2267) (-6.7077, 3.2128) (-6.7073, 3.203) (-6.7071, 3.1978) knots 0 0 0 0 0.152342 0.285545 0.405068 0.516839 0.624561 0.739342 0.861447 1 1 1 1
  spline S90 degree 3 poles (-6.7071, 3.1978) (-6.7073, 3.1936) (-6.7077, 3.1854) (-6.7117, 3.1739) (-6.7177, 3.1631) (-6.7261, 3.1538) (-6.7361, 3.1457) (-6.7472, 3.1399) (-6.7593, 3.1363) (-6.7676, 3.1359) (-6.7719, 3.1357) knots 0 0 0 0 0.123971 0.246778 0.365389 0.494204 0.623565 0.750071 0.871557 1 1 1 1
  spline S91 degree 3 poles (-6.7719, 3.1357) (-6.7753, 3.1355) (-6.7819, 3.1352) (-6.7914, 3.1327) (-6.7999, 3.1284) (-6.8073, 3.1225) (-6.8137, 3.1154) (-6.8181, 3.1071) (-6.821, 3.098) (-6.8213, 3.0917) (-6.8214, 3.0884) knots 0 0 0 0 0.13474 0.258614 0.382591 0.505187 0.629267 0.752001 0.871073 1 1 1 1
  line L75 (-6.8214, 3.0884) -> (-6.8214, 2.7839)
  spline S92 degree 3 poles (-6.8214, 2.7839) (-6.8214, 2.781) (-6.8213, 2.7757) (-6.8179, 2.7691) (-6.8124, 2.7646) (-6.8078, 2.7644) (-6.8054, 2.7643) knots 0 0 0 0 0.302016 0.536312 0.750494 1 1 1 1
  spline S93 degree 3 poles (-6.8054, 2.7643) (-6.8024, 2.7648) (-6.795, 2.7659) (-6.7892, 2.7706) (-6.7857, 2.7734) knots 0 0 0 0 0.406145 1 1 1 1
  line L76 (-6.7857, 2.7734) -> (-6.1875, 3.2319)
  line L77 (-6.525, 4.0446) -> (-6.7826, 3.9116)
  spline S94 degree 3 poles (-6.7826, 3.9116) (-6.7887, 3.9083) (-6.8002, 3.902) (-6.8131, 3.8872) (-6.8207, 3.869) (-6.8212, 3.856) (-6.8214, 3.8491) knots 0 0 0 0 0.262753 0.501306 0.739158 1 1 1 1
  line L78 (-6.8214, 3.8491) -> (-6.8214, 3.6161)
  spline S95 degree 3 poles (-6.8214, 3.6161) (-6.8216, 3.6117) (-6.822, 3.6032) (-6.8258, 3.5909) (-6.8316, 3.5795) (-6.84, 3.5695) (-6.8495, 3.5606) (-6.8608, 3.5546) (-6.8728, 3.5505) (-6.8814, 3.5502) (-6.8857, 3.55) knots 0 0 0 0 0.126957 0.249782 0.372684 0.501426 0.62965 0.751659 0.873043 1 1 1 1
  spline S96 degree 3 poles (-6.8857, 3.55) (-6.8901, 3.5502) (-6.8986, 3.5505) (-6.9106, 3.5546) (-6.9219, 3.5606) (-6.9314, 3.5695) (-6.9399, 3.5793) (-6.9456, 3.5907) (-6.9495, 3.6028) (-6.9498, 3.6113) (-6.95, 3.6156) knots 0 0 0 0 0.127439 0.249283 0.371755 0.500466 0.627999 0.751368 0.872561 1 1 1 1
  line L79 (-6.95, 3.6156) -> (-6.95, 3.8556)
  spline S97 degree 3 poles (-6.95, 3.8556) (-6.9497, 3.8634) (-6.949, 3.8792) (-6.9429, 3.9029) (-6.9337, 3.9269) (-6.9212, 3.9506) (-6.9067, 3.9726) (-6.891, 3.9916) (-6.8746, 4.0072) (-6.8623, 4.0146) (-6.8565, 4.0181) knots 0 0 0 0 0.119524 0.243206 0.374508 0.515457 0.654341 0.779636 0.894797 1 1 1 1
  line L80 (-6.8565, 4.0181) -> (-6.5746, 4.1636)
  spline S98 degree 3 poles (-6.5746, 4.1636) (-6.5644, 4.1681) (-6.5445, 4.177) (-6.5132, 4.186) (-6.4816, 4.1919) (-6.4604, 4.1925) (-6.4498, 4.1929) knots 0 0 0 0 0.256397 0.506809 0.754246 1 1 1 1
  spline S99 degree 3 poles (-6.4498, 4.1929) (-6.4384, 4.1925) (-6.4162, 4.1919) (-6.3841, 4.1867) (-6.3543, 4.1782) (-6.3361, 4.1695) (-6.3272, 4.1652) knots 0 0 0 0 0.269644 0.524554 0.766799 1 1 1 1
  line L81 (-6.3272, 4.1652) -> (-6.0482, 4.0181)
  spline S100 degree 3 poles (-6.0482, 4.0181) (-6.0418, 4.0142) (-6.0287, 4.0065) (-6.011, 3.991) (-5.9942, 3.9732) (-5.9791, 3.9527) (-5.9663, 3.931) (-5.9571, 3.9089) (-5.951, 3.8873) (-5.9503, 3.8729) (-5.95, 3.8658) knots 0 0 0 0 0.119157 0.241726 0.37148 0.508504 0.645292 0.77099 0.888372 1 1 1 1
  line L82 (-5.95, 3.8658) -> (-5.95, 3.6138)
  spline S101 degree 3 poles (-5.95, 3.6138) (-5.9502, 3.6096) (-5.9505, 3.6012) (-5.9543, 3.5892) (-5.9602, 3.5781) (-5.9685, 3.5685) (-5.9782, 3.5602) (-5.9893, 3.5544) (-6.0012, 3.5505) (-6.0094, 3.5502) (-6.0136, 3.55) knots 0 0 0 0 0.12765 0.251158 0.372942 0.501195 0.629448 0.753198 0.874572 1 1 1 1
  spline S102 degree 3 poles (-6.0136, 3.55) (-6.0179, 3.5502) (-6.0263, 3.5505) (-6.0383, 3.5544) (-6.0495, 3.5602) (-6.0594, 3.5685) (-6.068, 3.5781) (-6.074, 3.5893) (-6.0781, 3.6014) (-6.0784, 3.6098) (-6.0786, 3.6141) knots 0 0 0 0 0.126235 0.248374 0.370753 0.49928 0.627542 0.75097 0.873765 1 1 1 1
  line L83 (-6.0786, 3.6141) -> (-6.0786, 3.8585)
  spline S103 degree 3 poles (-6.0786, 3.8585) (-6.0787, 3.8634) (-6.0791, 3.8732) (-6.086, 3.8869) (-6.0973, 3.899) (-6.1072, 3.9047) (-6.1125, 3.9078) knots 0 0 0 0 0.230337 0.460431 0.709763 1 1 1 1
  line L84 (-6.1125, 3.9078) -> (-6.375, 4.0467)
  spline S104 degree 3 poles (-6.375, 4.0467) (-6.3803, 4.0493) (-6.3911, 4.0546) (-6.4088, 4.0597) (-6.4278, 4.0632) (-6.4408, 4.0639) (-6.4475, 4.0643) knots 0 0 0 0 0.234765 0.479498 0.732423 1 1 1 1
  spline S105 degree 3 poles (-6.4475, 4.0643) (-6.4546, 4.0637) (-6.4684, 4.0627) (-6.4885, 4.0589) (-6.5074, 4.0529) (-6.5192, 4.0474) (-6.525, 4.0446) knots 0 0 0 0 0.264576 0.515798 0.760431 1 1 1 1
  spline S106 degree 3 poles (-3.5386, 3.2007) (-3.5384, 3.2049) (-3.5381, 3.2134) (-3.534, 3.2253) (-3.5279, 3.2364) (-3.5194, 3.246) (-3.5095, 3.254) (-3.4983, 3.2599) (-3.4863, 3.2637) (-3.4779, 3.2641) (-3.4736, 3.2643) knots 0 0 0 0 0.126655 0.249859 0.371763 0.500453 0.628013 0.750799 0.873345 1 1 1 1
  spline S107 degree 3 poles (-3.4736, 3.2643) (-3.4694, 3.2641) (-3.4612, 3.2638) (-3.4493, 3.2599) (-3.4382, 3.2541) (-3.4285, 3.246) (-3.4202, 3.2363) (-3.4144, 3.2251) (-3.4105, 3.2131) (-3.4102, 3.2047) (-3.41, 3.2004) knots 0 0 0 0 0.12536 0.246668 0.370351 0.497111 0.625295 0.748978 0.872419 1 1 1 1
  line L85 (-3.41, 3.2004) -> (-3.41, 2.9487)
  spline S108 degree 3 poles (-3.41, 2.9487) (-3.4105, 2.9404) (-3.4114, 2.9239) (-3.4178, 2.8995) (-3.4277, 2.8754) (-3.4413, 2.8524) (-3.4573, 2.8308) (-3.4752, 2.8119) (-3.4947, 2.7959) (-3.5091, 2.7879) (-3.5163, 2.7839) knots 0 0 0 0 0.120295 0.241539 0.367541 0.499794 0.632883 0.759219 0.880834 1 1 1 1
  line L86 (-3.5163, 2.7839) -> (-3.7685, 2.6574)
  spline S109 degree 3 poles (-3.7685, 2.6574) (-3.7799, 2.6519) (-3.8025, 2.6411) (-3.8381, 2.6297) (-3.8745, 2.6227) (-3.899, 2.6219) (-3.9113, 2.6214) knots 0 0 0 0 0.255305 0.504536 0.751856 1 1 1 1
  spline S110 degree 3 poles (-3.9113, 2.6214) (-3.923, 2.6219) (-3.9466, 2.6229) (-3.9822, 2.6306) (-4.0184, 2.6422) (-4.0416, 2.6537) (-4.0535, 2.6596) knots 0 0 0 0 0.234952 0.477147 0.731798 1 1 1 1
  line L87 (-4.0535, 2.6596) -> (-4.3035, 2.7868)
  spline S111 degree 3 poles (-4.3035, 2.7868) (-4.3113, 2.7911) (-4.3269, 2.7995) (-4.3474, 2.8161) (-4.3657, 2.835) (-4.3812, 2.8564) (-4.3941, 2.8796) (-4.4032, 2.9045) (-4.4091, 2.9308) (-4.4097, 2.9487) (-4.41, 2.9578) knots 0 0 0 0 0.125475 0.2491 0.371934 0.496998 0.621836 0.746394 0.871303 1 1 1 1
  line L88 (-4.41, 2.9578) -> (-4.41, 3.2007)
  spline S112 degree 3 poles (-4.41, 3.2007) (-4.4098, 3.2049) (-4.4094, 3.2133) (-4.4057, 3.2254) (-4.3995, 3.2363) (-4.3913, 3.246) (-4.3816, 3.254) (-4.3707, 3.2599) (-4.3588, 3.2637) (-4.3506, 3.2641) (-4.3464, 3.2643) knots 0 0 0 0 0.127946 0.25174 0.374887 0.503437 0.63056 0.752626 0.874282 1 1 1 1
  spline S113 degree 3 poles (-4.3464, 3.2643) (-4.3421, 3.2641) (-4.3337, 3.2638) (-4.3217, 3.2598) (-4.3103, 3.2544) (-4.3005, 3.2462) (-4.2918, 3.2369) (-4.2861, 3.2258) (-4.2819, 3.2141) (-4.2816, 3.2058) (-4.2814, 3.2016) knots 0 0 0 0 0.127432 0.250729 0.375227 0.50357 0.631371 0.752946 0.874787 1 1 1 1
  line L89 (-4.2814, 3.2016) -> (-4.2814, 3.1357)
  line L90 (-4.2814, 3.1357) -> (-3.5386, 3.1357)
  line L91 (-3.5386, 3.1357) -> (-3.5386, 3.2007)
  spline S114 degree 3 poles (-1.1075, 4.1605) (-1.1003, 4.1654) (-1.0863, 4.175) (-1.0632, 4.1854) (-1.0391, 4.1917) (-1.0226, 4.1925) (-1.0144, 4.1929) knots 0 0 0 0 0.259405 0.508544 0.754257 1 1 1 1
  spline S115 degree 3 poles (-1.0144, 4.1929) (-1.005, 4.1923) (-0.9864, 4.1913) (-0.9595, 4.1835) (-0.9348, 4.1701) (-0.9125, 4.1522) (-0.8939, 4.1305) (-0.8799, 4.1063) (-0.8714, 4.0797) (-0.8705, 4.0612) (-0.87, 4.0518) knots 0 0 0 0 0.126245 0.24873 0.371883 0.501018 0.62976 0.75261 0.873755 1 1 1 1
  line L92 (-0.87, 4.0518) -> (-0.87, 3.729)
  spline S116 degree 3 poles (-0.87, 3.729) (-0.8706, 3.7192) (-0.8717, 3.6993) (-0.8824, 3.6704) (-0.8988, 3.6426) (-0.9173, 3.6208) (-0.9346, 3.6047) (-0.9485, 3.5937) (-0.9634, 3.5849) (-0.9787, 3.5772) (-0.9948, 3.5713) (-1.0116, 3.5674) (-1.0291, 3.5648) (-1.041, 3.5645) (-1.047, 3.5643) knots 0 0 0 0 0.110459 0.223148 0.342644 0.474148 0.54296 0.6087 0.673406 0.737899 0.801293 0.865961 0.932005 1 1 1 1
  spline S117 degree 3 poles (-1.047, 3.5643) (-1.0514, 3.5646) (-1.0601, 3.5651) (-1.0727, 3.5689) (-1.084, 3.5759) (-1.0939, 3.5851) (-1.1023, 3.5955) (-1.1085, 3.6069) (-1.1123, 3.619) (-1.1127, 3.6273) (-1.1129, 3.6315) knots 0 0 0 0 0.127348 0.250965 0.376177 0.506901 0.638364 0.760387 0.87927 1 1 1 1
  spline S118 degree 3 poles (-1.1129, 3.6315) (-1.1127, 3.6369) (-1.1125, 3.6469) (-1.1097, 3.6607) (-1.1048, 3.6717) (-1.0977, 3.6806) (-1.0874, 3.6868) (-1.0748, 3.6929) (-1.0586, 3.6983) (-1.0404, 3.7029) (-1.0226, 3.7084) (-1.0085, 3.7187) (-1, 3.7328) (-0.999, 3.7434) (-0.9986, 3.7489) knots 0 0 0 0 0.089812 0.165231 0.230095 0.287663 0.349673 0.426046 0.519675 0.62936 0.736624 0.826058 0.910331 1 1 1 1
  line L93 (-0.9986, 3.7489) -> (-0.9986, 4.0431)
  spline S119 degree 3 poles (-0.9986, 4.0431) (-0.9986, 4.0462) (-0.9988, 4.0518) (-1.0018, 4.0588) (-1.0067, 4.0637) (-1.011, 4.0641) (-1.0133, 4.0643) knots 0 0 0 0 0.323315 0.566859 0.773057 1 1 1 1
  spline S120 degree 3 poles (-1.0133, 4.0643) (-1.0167, 4.0639) (-1.0245, 4.0631) (-1.0309, 4.0583) (-1.0345, 4.0556) knots 0 0 0 0 0.42835 1 1 1 1
  line L94 (-1.0345, 4.0556) -> (-1.6325, 3.5973)
  spline S121 degree 3 poles (-1.6325, 3.5973) (-1.6397, 3.5922) (-1.6538, 3.5822) (-1.6773, 3.5721) (-1.7015, 3.5653) (-1.7179, 3.5646) (-1.7263, 3.5643) knots 0 0 0 0 0.261351 0.512303 0.754244 1 1 1 1
  spline S122 degree 3 poles (-1.7263, 3.5643) (-1.7355, 3.5647) (-1.7539, 3.5656) (-1.7804, 3.5735) (-1.805, 3.5863) (-1.8271, 3.6038) (-1.8458, 3.6241) (-1.86, 3.6461) (-1.8684, 3.6698) (-1.8695, 3.6861) (-1.87, 3.6942) knots 0 0 0 0 0.130284 0.257797 0.385118 0.519315 0.651174 0.771096 0.886275 1 1 1 1
  line L95 (-1.87, 3.6942) -> (-1.87, 4.0283)
  spline S123 degree 3 poles (-1.87, 4.0283) (-1.8698, 4.0338) (-1.8694, 4.0446) (-1.8669, 4.0604) (-1.8629, 4.0758) (-1.8571, 4.0906) (-1.8494, 4.1047) (-1.8402, 4.1184) (-1.8295, 4.1316) (-1.813, 4.1479) (-1.7908, 4.1656) (-1.7619, 4.1813) (-1.7315, 4.1911) (-1.7106, 4.1923) (-1.7001, 4.1929) knots 0 0 0 0 0.062642 0.124202 0.184472 0.245252 0.306591 0.369566 0.434735 0.502591 0.635605 0.760198 0.879447 1 1 1 1
  spline S124 degree 3 poles (-1.7001, 4.1929) (-1.6944, 4.1927) (-1.6836, 4.1923) (-1.6686, 4.1891) (-1.6557, 4.1841) (-1.6453, 4.1765) (-1.6368, 4.1671) (-1.6311, 4.1552) (-1.6277, 4.1414) (-1.6273, 4.1316) (-1.6271, 4.1263) knots 0 0 0 0 0.152342 0.285545 0.405068 0.516839 0.624561 0.739342 0.861447 1 1 1 1
  spline S125 degree 3 poles (-1.6271, 4.1263) (-1.6273, 4.1222) (-1.6277, 4.114) (-1.6317, 4.1024) (-1.6377, 4.0916) (-1.6461, 4.0823) (-1.6561, 4.0742) (-1.6672, 4.0685) (-1.6793, 4.0649) (-1.6876, 4.0645) (-1.6919, 4.0643) knots 0 0 0 0 0.123971 0.246778 0.365389 0.494204 0.623565 0.750071 0.871557 1 1 1 1
  spline S126 degree 3 poles (-1.6919, 4.0643) (-1.6953, 4.0641) (-1.7019, 4.0638) (-1.7114, 4.0612) (-1.7199, 4.057) (-1.7273, 4.0511) (-1.7337, 4.044) (-1.7381, 4.0357) (-1.741, 4.0266) (-1.7413, 4.0203) (-1.7414, 4.017) knots 0 0 0 0 0.13474 0.258614 0.382591 0.505187 0.629267 0.752001 0.871073 1 1 1 1
  line L96 (-1.7414, 4.017) -> (-1.7414, 3.7125)
  spline S127 degree 3 poles (-1.7414, 3.7125) (-1.7414, 3.7095) (-1.7413, 3.7043) (-1.7379, 3.6977) (-1.7324, 3.6931) (-1.7278, 3.693) (-1.7254, 3.6929) knots 0 0 0 0 0.302016 0.536312 0.750494 1 1 1 1
  spline S128 degree 3 poles (-1.7254, 3.6929) (-1.7224, 3.6933) (-1.715, 3.6945) (-1.7092, 3.6992) (-1.7057, 3.702) knots 0 0 0 0 0.406145 1 1 1 1
  line L97 (-1.7057, 3.702) -> (-1.1075, 4.1605)
  spline S129 degree 3 poles (-1.87, 2.2714) (-1.8698, 2.2759) (-1.8695, 2.2846) (-1.8657, 2.297) (-1.8595, 2.3081) (-1.8514, 2.3179) (-1.8414, 2.3257) (-1.8304, 2.3317) (-1.8181, 2.3351) (-1.8096, 2.3355) (-1.8053, 2.3357) knots 0 0 0 0 0.132059 0.255591 0.378303 0.504399 0.627717 0.749385 0.872312 1 1 1 1
  spline S130 degree 3 poles (-1.8053, 2.3357) (-1.8014, 2.3356) (-1.7934, 2.3352) (-1.7858, 2.3332) (-1.7818, 2.3321) knots 0 0 0 0 0.489728 1 1 1 1
  line L98 (-1.7818, 2.3321) -> (-0.9164, 2.0908)
  spline S131 degree 3 poles (-0.9164, 2.0908) (-0.9127, 2.0896) (-0.9056, 2.0871) (-0.8962, 2.0815) (-0.8879, 2.0754) (-0.8814, 2.0678) (-0.8762, 2.0593) (-0.8726, 2.0496) (-0.8703, 2.039) (-0.8701, 2.0316) (-0.87, 2.0277) knots 0 0 0 0 0.138313 0.265623 0.385651 0.501271 0.618171 0.736456 0.862919 1 1 1 1
  spline S132 degree 3 poles (-0.87, 2.0277) (-0.8704, 2.0206) (-0.8712, 2.0074) (-0.8786, 1.9893) (-0.8922, 1.9761) (-0.9036, 1.9716) (-0.9095, 1.9692) knots 0 0 0 0 0.277202 0.519882 0.749783 1 1 1 1
  line L99 (-0.9095, 1.9692) -> (-1.7879, 1.7243)
  spline S133 degree 3 poles (-1.7879, 1.7243) (-1.791, 1.7235) (-1.7972, 1.7218) (-1.8035, 1.7215) (-1.8066, 1.7214) knots 0 0 0 0 0.517816 1 1 1 1
  spline S134 degree 3 poles (-1.8066, 1.7214) (-1.8109, 1.7216) (-1.8192, 1.722) (-1.8312, 1.7255) (-1.8419, 1.7315) (-1.8517, 1.7392) (-1.8596, 1.7484) (-1.8657, 1.7585) (-1.8694, 1.7694) (-1.8698, 1.777) (-1.87, 1.7808) knots 0 0 0 0 0.132938 0.258677 0.385506 0.51613 0.64465 0.76339 0.880942 1 1 1 1
  spline S135 degree 3 poles (-1.87, 1.7808) (-1.8699, 1.7848) (-1.8697, 1.7923) (-1.8674, 1.803) (-1.8639, 1.8127) (-1.8589, 1.8213) (-1.8526, 1.8289) (-1.8445, 1.8349) (-1.8353, 1.8402) (-1.8283, 1.8425) (-1.8247, 1.8437) knots 0 0 0 0 0.140927 0.268493 0.390294 0.506862 0.621754 0.739105 0.863907 1 1 1 1
  line L100 (-1.8247, 1.8437) -> (-1.6557, 1.8906)
  line L101 (-1.6557, 1.8906) -> (-1.6557, 2.1663)
  line L102 (-1.6557, 2.1663) -> (-1.8376, 2.2163)
  spline S136 degree 3 poles (-1.8376, 2.2163) (-1.8396, 2.2169) (-1.8438, 2.2181) (-1.8495, 2.2222) (-1.8547, 2.2281) (-1.8615, 2.2379) (-1.8685, 2.2523) (-1.8695, 2.265) (-1.87, 2.2714) knots 0 0 0 0 0.090571 0.190093 0.306571 0.438985 0.717416 1 1 1 1
  spline S137 degree 3 poles (-3.6475, 4.1605) (-3.6403, 4.1654) (-3.6263, 4.175) (-3.6032, 4.1854) (-3.5791, 4.1917) (-3.5626, 4.1925) (-3.5544, 4.1929) knots 0 0 0 0 0.259405 0.508544 0.754257 1 1 1 1
  spline S138 degree 3 poles (-3.5544, 4.1929) (-3.545, 4.1923) (-3.5264, 4.1913) (-3.4995, 4.1835) (-3.4748, 4.1701) (-3.4525, 4.1522) (-3.4339, 4.1305) (-3.4199, 4.1063) (-3.4114, 4.0797) (-3.4105, 4.0612) (-3.41, 4.0518) knots 0 0 0 0 0.126245 0.24873 0.371883 0.501018 0.62976 0.75261 0.873755 1 1 1 1
  line L103 (-3.41, 4.0518) -> (-3.41, 3.729)
  spline S139 degree 3 poles (-3.41, 3.729) (-3.4106, 3.7192) (-3.4117, 3.6993) (-3.4224, 3.6704) (-3.4388, 3.6426) (-3.4573, 3.6208) (-3.4746, 3.6047) (-3.4885, 3.5937) (-3.5034, 3.5849) (-3.5187, 3.5772) (-3.5348, 3.5713) (-3.5516, 3.5674) (-3.5691, 3.5648) (-3.581, 3.5645) (-3.587, 3.5643) knots 0 0 0 0 0.110459 0.223148 0.342644 0.474148 0.54296 0.6087 0.673406 0.737899 0.801293 0.865961 0.932005 1 1 1 1
  spline S140 degree 3 poles (-3.587, 3.5643) (-3.5914, 3.5646) (-3.6001, 3.5651) (-3.6127, 3.5689) (-3.624, 3.5759) (-3.6339, 3.5851) (-3.6423, 3.5955) (-3.6485, 3.6069) (-3.6523, 3.619) (-3.6527, 3.6273) (-3.6529, 3.6315) knots 0 0 0 0 0.127348 0.250965 0.376177 0.506901 0.638364 0.760387 0.87927 1 1 1 1
  spline S141 degree 3 poles (-3.6529, 3.6315) (-3.6527, 3.6369) (-3.6525, 3.6469) (-3.6497, 3.6607) (-3.6448, 3.6717) (-3.6377, 3.6806) (-3.6274, 3.6868) (-3.6148, 3.6929) (-3.5986, 3.6983) (-3.5804, 3.7029) (-3.5626, 3.7084) (-3.5485, 3.7187) (-3.54, 3.7328) (-3.539, 3.7434) (-3.5386, 3.7489) knots 0 0 0 0 0.089812 0.165231 0.230095 0.287663 0.349673 0.426046 0.519675 0.62936 0.736624 0.826058 0.910331 1 1 1 1
  line L104 (-3.5386, 3.7489) -> (-3.5386, 4.0431)
  spline S142 degree 3 poles (-3.5386, 4.0431) (-3.5386, 4.0462) (-3.5388, 4.0518) (-3.5418, 4.0588) (-3.5467, 4.0637) (-3.551, 4.0641) (-3.5533, 4.0643) knots 0 0 0 0 0.323315 0.566859 0.773057 1 1 1 1
  spline S143 degree 3 poles (-3.5533, 4.0643) (-3.5567, 4.0639) (-3.5645, 4.0631) (-3.5709, 4.0583) (-3.5745, 4.0556) knots 0 0 0 0 0.42835 1 1 1 1
  line L105 (-3.5745, 4.0556) -> (-4.1725, 3.5973)
  spline S144 degree 3 poles (-4.1725, 3.5973) (-4.1797, 3.5922) (-4.1938, 3.5822) (-4.2173, 3.5721) (-4.2415, 3.5653) (-4.2579, 3.5646) (-4.2663, 3.5643) knots 0 0 0 0 0.261351 0.512303 0.754244 1 1 1 1
  spline S145 degree 3 poles (-4.2663, 3.5643) (-4.2755, 3.5647) (-4.2939, 3.5656) (-4.3204, 3.5735) (-4.345, 3.5863) (-4.3671, 3.6038) (-4.3858, 3.6241) (-4.4, 3.6461) (-4.4084, 3.6698) (-4.4095, 3.6861) (-4.41, 3.6942) knots 0 0 0 0 0.130284 0.257797 0.385118 0.519315 0.651174 0.771096 0.886275 1 1 1 1
  line L106 (-4.41, 3.6942) -> (-4.41, 4.0283)
  spline S146 degree 3 poles (-4.41, 4.0283) (-4.4098, 4.0338) (-4.4094, 4.0446) (-4.4069, 4.0604) (-4.4029, 4.0758) (-4.3971, 4.0906) (-4.3894, 4.1047) (-4.3802, 4.1184) (-4.3695, 4.1316) (-4.353, 4.1479) (-4.3308, 4.1656) (-4.3019, 4.1813) (-4.2715, 4.1911) (-4.2506, 4.1923) (-4.2401, 4.1929) knots 0 0 0 0 0.062642 0.124202 0.184472 0.245252 0.306591 0.369566 0.434735 0.502591 0.635605 0.760198 0.879447 1 1 1 1
  spline S147 degree 3 poles (-4.2401, 4.1929) (-4.2344, 4.1927) (-4.2236, 4.1923) (-4.2086, 4.1891) (-4.1957, 4.1841) (-4.1853, 4.1765) (-4.1768, 4.1671) (-4.1711, 4.1552) (-4.1677, 4.1414) (-4.1673, 4.1316) (-4.1671, 4.1263) knots 0 0 0 0 0.152342 0.285545 0.405068 0.516839 0.624561 0.739342 0.861447 1 1 1 1
  spline S148 degree 3 poles (-4.1671, 4.1263) (-4.1673, 4.1222) (-4.1677, 4.114) (-4.1717, 4.1024) (-4.1777, 4.0916) (-4.1861, 4.0823) (-4.1961, 4.0742) (-4.2072, 4.0685) (-4.2193, 4.0649) (-4.2276, 4.0645) (-4.2319, 4.0643) knots 0 0 0 0 0.123971 0.246778 0.365389 0.494204 0.623565 0.750071 0.871557 1 1 1 1
  spline S149 degree 3 poles (-4.2319, 4.0643) (-4.2353, 4.0641) (-4.2419, 4.0638) (-4.2514, 4.0612) (-4.2599, 4.057) (-4.2673, 4.0511) (-4.2737, 4.044) (-4.2781, 4.0357) (-4.281, 4.0266) (-4.2813, 4.0203) (-4.2814, 4.017) knots 0 0 0 0 0.13474 0.258614 0.382591 0.505187 0.629267 0.752001 0.871073 1 1 1 1
  line L107 (-4.2814, 4.017) -> (-4.2814, 3.7125)
  spline S150 degree 3 poles (-4.2814, 3.7125) (-4.2814, 3.7095) (-4.2813, 3.7043) (-4.2779, 3.6977) (-4.2724, 3.6931) (-4.2678, 3.693) (-4.2654, 3.6929) knots 0 0 0 0 0.302016 0.536312 0.750494 1 1 1 1
  spline S151 degree 3 poles (-4.2654, 3.6929) (-4.2624, 3.6933) (-4.255, 3.6945) (-4.2492, 3.6992) (-4.2457, 3.702) knots 0 0 0 0 0.406145 1 1 1 1
  line L108 (-4.2457, 3.702) -> (-3.6475, 4.1605)
  spline S152 degree 3 poles (-0.9986, 3.2007) (-0.9984, 3.2049) (-0.9981, 3.2134) (-0.994, 3.2253) (-0.9879, 3.2364) (-0.9794, 3.246) (-0.9695, 3.254) (-0.9583, 3.2599) (-0.9463, 3.2637) (-0.9379, 3.2641) (-0.9336, 3.2643) knots 0 0 0 0 0.126655 0.249859 0.371763 0.500453 0.628013 0.750799 0.873345 1 1 1 1
  spline S153 degree 3 poles (-0.9336, 3.2643) (-0.9294, 3.2641) (-0.9212, 3.2638) (-0.9093, 3.2599) (-0.8982, 3.2541) (-0.8885, 3.246) (-0.8802, 3.2363) (-0.8744, 3.2251) (-0.8705, 3.2131) (-0.8702, 3.2047) (-0.87, 3.2004) knots 0 0 0 0 0.12536 0.246668 0.370351 0.497111 0.625295 0.748978 0.872419 1 1 1 1
  line L109 (-0.87, 3.2004) -> (-0.87, 2.9487)
  spline S154 degree 3 poles (-0.87, 2.9487) (-0.8705, 2.9404) (-0.8714, 2.9239) (-0.8778, 2.8995) (-0.8877, 2.8754) (-0.9013, 2.8524) (-0.9173, 2.8308) (-0.9352, 2.8119) (-0.9547, 2.7959) (-0.9691, 2.7879) (-0.9763, 2.7839) knots 0 0 0 0 0.120295 0.241539 0.367541 0.499794 0.632883 0.759219 0.880834 1 1 1 1
  line L110 (-0.9763, 2.7839) -> (-1.2285, 2.6574)
  spline S155 degree 3 poles (-1.2285, 2.6574) (-1.2399, 2.6519) (-1.2625, 2.6411) (-1.2981, 2.6297) (-1.3345, 2.6227) (-1.359, 2.6219) (-1.3713, 2.6214) knots 0 0 0 0 0.255305 0.504536 0.751856 1 1 1 1
  spline S156 degree 3 poles (-1.3713, 2.6214) (-1.383, 2.6219) (-1.4066, 2.6229) (-1.4422, 2.6306) (-1.4784, 2.6422) (-1.5016, 2.6537) (-1.5135, 2.6596) knots 0 0 0 0 0.234952 0.477147 0.731798 1 1 1 1
  line L111 (-1.5135, 2.6596) -> (-1.7635, 2.7868)
  spline S157 degree 3 poles (-1.7635, 2.7868) (-1.7713, 2.7911) (-1.7869, 2.7995) (-1.8074, 2.8161) (-1.8257, 2.835) (-1.8412, 2.8564) (-1.8541, 2.8796) (-1.8632, 2.9045) (-1.8691, 2.9308) (-1.8697, 2.9487) (-1.87, 2.9578) knots 0 0 0 0 0.125475 0.2491 0.371934 0.496998 0.621836 0.746394 0.871303 1 1 1 1
  line L112 (-1.87, 2.9578) -> (-1.87, 3.2007)
  spline S158 degree 3 poles (-1.87, 3.2007) (-1.8698, 3.2049) (-1.8694, 3.2133) (-1.8657, 3.2254) (-1.8595, 3.2363) (-1.8513, 3.246) (-1.8416, 3.254) (-1.8307, 3.2599) (-1.8188, 3.2637) (-1.8106, 3.2641) (-1.8064, 3.2643) knots 0 0 0 0 0.127946 0.25174 0.374887 0.503437 0.63056 0.752626 0.874282 1 1 1 1
  spline S159 degree 3 poles (-1.8064, 3.2643) (-1.8021, 3.2641) (-1.7937, 3.2638) (-1.7817, 3.2598) (-1.7703, 3.2544) (-1.7605, 3.2462) (-1.7518, 3.2369) (-1.7461, 3.2258) (-1.7419, 3.2141) (-1.7416, 3.2058) (-1.7414, 3.2016) knots 0 0 0 0 0.127432 0.250729 0.375227 0.50357 0.631371 0.752946 0.874787 1 1 1 1
  line L113 (-1.7414, 3.2016) -> (-1.7414, 3.1357)
  line L114 (-1.7414, 3.1357) -> (-0.9986, 3.1357)
  line L115 (-0.9986, 3.1357) -> (-0.9986, 3.2007)
  spline S160 degree 3 poles (-3.5026, 2.1741) (-3.4953, 2.1702) (-3.4811, 2.1625) (-3.462, 2.1487) (-3.4458, 2.1329) (-3.4328, 2.1152) (-3.4223, 2.0961) (-3.4153, 2.075) (-3.4106, 2.0524) (-3.4102, 2.0366) (-3.41, 2.0286) knots 0 0 0 0 0.136027 0.26437 0.385998 0.504571 0.622472 0.742449 0.868049 1 1 1 1
  spline S161 degree 3 poles (-3.41, 2.0286) (-3.4102, 2.0204) (-3.4106, 2.0046) (-3.4153, 1.9818) (-3.4223, 1.9606) (-3.4328, 1.9415) (-3.4458, 1.924) (-3.462, 1.9085) (-3.4811, 1.8948) (-3.4953, 1.8875) (-3.5026, 1.8837) knots 0 0 0 0 0.133344 0.260309 0.380444 0.4985 0.616252 0.737186 0.864982 1 1 1 1